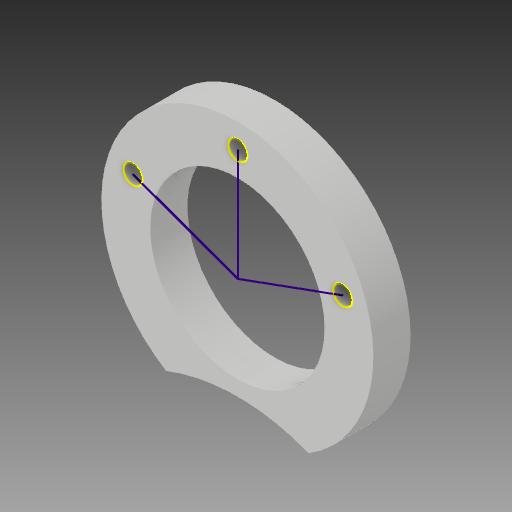
# Autodesk Inventor part: 円 46.9mm
Saved by Autodesk Inventor 2019 (Build 230136000, 136)
## iProperties
Created: 2020-09-27
Part Number: 円 46.9mm
Material: 一般
Document SubType Name: Modeling
Designer: Toshihito
Density: 1 g/cm^3
Appearance: 既定
Author: Toshihito
Autodesk Inventor part; units mm, degrees
ref_plane "YZ Plane" through (0, 0, 0) normal (1, 0, 0) x (0, 1, 0)
ref_plane "XZ Plane" through (0, 0, 0) normal (0, 1, 0) x (-1, 0, 0)
ref_plane "XY Plane" through (0, 0, 0) normal (0, 0, 1) x (1, 0, 0)
sketch "スケッチ1" plane through (0, 0, 0) normal (0, 0, 1) x (1, 0, 0)
  circle A0 centre (0, 0) radius 23.45
  circle A1 centre (0, 0) radius 36.55
  line L0 (0, 0) -> (-28.1908, 10.2606) construction
  line L1 (0, 0) -> (28.1908, 10.2606) construction
  line L2 (-39.5959, 0) -> (43.1917, 0) construction
  line L3 (0, 0) -> (0, 30) construction
  circle A2 centre (-28.1908, 10.2606) radius 2.55
  circle A3 centre (0, 30) radius 2.55
  circle A4 centre (28.1908, 10.2606) radius 2.55
  dimension "d0" = 73.1
  dimension "d1" = 46.9
  dimension "d2" = 30
  dimension "d3" = 30
  dimension "d6" = 20
  dimension "d7" = 20
  dimension "d8" = 30
  dimension "d9" = 5.1
  dimension "d10" = 5.1
  dimension "d11" = 5.1
  constraints: 8 end point, 5 centre point, 5 coincident, 1 horizontal, 1 vertical
  measures "d0" diameter of A1
  measures "d1" diameter of A0
  measures "d2" distance of L0.start L0.end
  measures "d3" distance of L0.start L1.end
  measures "d6" angle of L2 L0
  measures "d7" angle of L2 L1
  measures "d8" distance of L0.start L3.end
  measures "d9" diameter of A2
  measures "d10" diameter of A3
  measures "d11" diameter of A4
extrude "押し出し1" add sketch "スケッチ1" along normal blind 10
sketch "スケッチ2" plane through (0, 0, 10) normal (0, 0, 1) x (1, 0, 0)
  line L0 (0, 0) -> (0, -80) construction
  circle A0 centre (0, -80) radius 52.5
  dimension "d14" = 80
  dimension "d18" = 105
  constraints: 2 end point, 1 centre point, 1 vertical
  measures "d14" distance of L0.start L0.end
  measures "d18" diameter of A0
extrude "押し出し2" cut sketch "スケッチ2" against normal blind 10
sketch "スケッチ3" plane through (0, 0, 10) normal (0, 0, 1) x (1, 0, 0)
  circle A0 centre (28.1908, 10.2606) radius 2.55 projected
  line L0 (0, 0) -> (28.1908, 10.2606)
  circle A1 centre (-28.1908, 10.2606) radius 2.55 projected
  line L1 (-28.1908, 10.2606) -> (0, 0)
  circle A2 centre (0, 30) radius 2.55 projected
  line L2 (0, 0) -> (0, 30)
  constraints: 6 end point, 1 vertical
